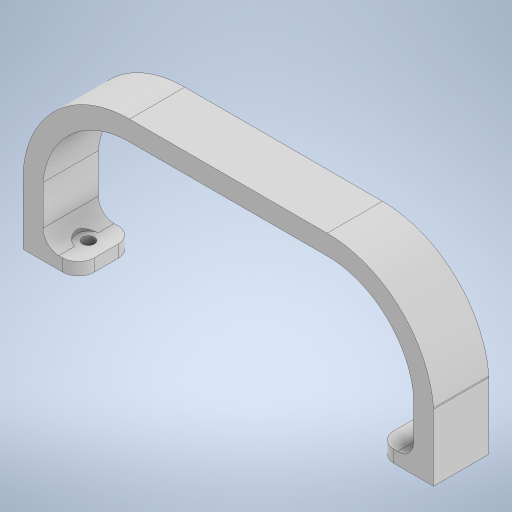
# Autodesk Inventor part: antenna_mount_v2
Saved by Autodesk Inventor 2024 (Build 280153000, 153)
## iProperties
Created: 2024-05-01
Part Number: antenna_mount_v2
Material: Generic
Document SubType Name: Modeling
Designer: Jacob
Density: 1 g/cm^3
Appearance: Default
Author: Jacob
## iProperties of the stored document antenna_mount_v2_3DPrint.ipt
Created: 2024-05-01
Part Number: antenna_mount_v2_3DPrint
Material: Generic
Document SubType Name: Modeling
Designer: Jacob
Density: 1 g/cm^3
Appearance: Default
Author: Jacob
Autodesk Inventor part; units mm, degrees
ref_plane "YZ Plane" through (0, 0, 0) normal (1, 0, 0) x (0, 1, 0)
sketch "Sketch11" plane through (0, 0, 0) normal (0, 0, 1) x (1, 0, 0)
  line L0 (25, -2.5) -> (-25, -2.5)
  line L1 (-25, -2.5) -> (-25, 2.5)
  line L2 (-25, 2.5) -> (25, 2.5)
  line L3 (25, 2.5) -> (25, -2.5)
  line L4 (25, -2.5) -> (-25, 2.5) construction
  line L5 (-25, -2.5) -> (25, 2.5) construction
  line L6 (0, 0) -> (-52.5, 0)
  line L7 (0, 0) -> (52.5, 0)
  circle A0 centre (25, -24.5) radius 24.5
  line L8 (52.5, 0) -> (52.5, -27.0879)
  circle A1 centre (25, -24.5) radius 27
  circle A2 centre (25, -24.5) radius 22
  line L9 (0, -2.5) -> (0, -42.1682)
  circle A3 centre (-25, -24.5) radius 24.5
  circle A4 centre (-25, -24.5) radius 27
  circle A5 centre (-25, -24.5) radius 22
  line L10 (-25, -24.5) -> (-52, -24.5)
  line L11 (-25, -24.5) -> (52.5, -24.5)
  point P0 (25, 0)
  point P1 (-47, -24.5)
  point P2 (47, -24.5)
  point P3 (52, -24.5)
  dimension "d43" = 49
  dimension "d39" = 50
  dimension "d40" = 5
  dimension "d41" = 52.5
  dimension "d42" = 52.5
  constraints: 24 end point, 5 horizontal, 4 coincident, 4 midpoint, 3 symmetric about line, 3 vertical, 2 centre point, 2 parallel, 2 point on line, 1 perpendicular, 1 vertical alignment, 13 other
  measures "d39" distance of L1.end L2.end
  measures "d40" distance of L0.end L1.end
  measures "d41" distance of L6.start L6.end
  measures "d42" distance of L6.start L7.end
extrude "Extrusion9" add sketch "Sketch11" along normal blind 12.5 contours L0 A0 L3 | L3 A0 L11 A2 | L0 A1 L7 A0 | L7 A1 L3 | L3 A1 L7 | L7 A1 L11 A0 | L0 A4 L6 L7 A1 | A1 L7 L6 A4 L2 | A4 L6 L1 | L1 L6 A4 | L0 A3 L6 A4 | A3 L0 L1 | A3 L10 A4 L6 | L1 A5 L10 A3
ref_plane "Work Plane1" through (-25, -39.5, 0) normal (0, -1, 0) x (1, 0, 0)
sketch "Sketch12" plane through (-25, -39.5, 0) normal (0, -1, 0) x (1, 0, 0)
  line L0 (25, 0) -> (25, 12.5)
  line L1 (50, 12.5) -> (0, 12.5) projected
  line L2 (25, 6.25) -> (0, 6.25)
  line L3 (0, 6.25) -> (50, 6.25)
  line L4 (0, 6.25) -> (5, 6.25)
  line L5 (5, 6.25) -> (5, 12.5)
  line L6 (5, 12.5) -> (0, 12.5)
  line L7 (0, 12.5) -> (0, 6.25)
  line L8 (5, 6.25) -> (0, 6.25)
  line L9 (0, 6.25) -> (0, 0)
  line L10 (0, 0) -> (5, 0)
  line L11 (5, 0) -> (5, 6.25)
  line L12 (50, 6.25) -> (45, 6.25)
  line L13 (45, 6.25) -> (45, 12.5)
  line L14 (45, 12.5) -> (50, 12.5)
  line L15 (50, 12.5) -> (50, 6.25)
  line L16 (50, 0) -> (72, 0) projected
  line L17 (50, 6.25) -> (45, 6.25)
  line L18 (45, 6.25) -> (45, 0)
  line L19 (45, 0) -> (50, 0)
  line L20 (50, 0) -> (50, 6.25)
  point P0 (50, 0)
  point P1 (45, 6.25)
  point P2 (45, 6.25)
  dimension "d47" = 25
  dimension "d48" = 50
  dimension "d49" = 5
  dimension "d50" = 5
  constraints: 38 end point, 8 parallel, 6 point on line, 5 horizontal, 4 perpendicular, 2 midpoint
  measures "d47" distance of L2.start L2.end
  measures "d48" distance of L2.end L3.end
  measures "d49" distance of L6.end L5.end
  measures "d50" distance of L13.end L14.end
extrude "Extrusion10" add sketch "Sketch12" against normal up to surface (37 mm away) contours L11 L10 L9 L2 | L2 L7 L1 L5 | L13 L1 L15 L3 | L3 L20 L19 L18
sketch "Sketch13" plane through (-25, -39.5, 0) normal (-1, 0, 0) x (0, 0, 1)
  line L0 (0, 0) -> (12.5, 0) projected
  line L1 (0, 0) -> (0, 37) projected
  line L2 (12.5, 0) -> (0, 0)
  line L3 (0, 0) -> (0, 3)
  line L4 (0, 3) -> (12.5, 3)
  line L5 (12.5, 3) -> (12.5, 0)
  line L6 (0, 0) -> (12.5, 0)
  line L7 (12.5, 0) -> (12.5, 3)
  line L8 (12.5, 3) -> (0, 3)
  line L9 (0, 3) -> (0, 0)
  point P0 (0, 39.5)
  dimension "d53" = 3
  constraints: 16 end point, 4 parallel, 2 horizontal, 2 perpendicular, 1 point on line
  measures "d53" distance of L2.end L3.end
extrude "Extrusion11" add sketch "Sketch13" along normal blind 8.75
sketch "Sketch14" plane through (25, -39.5, 12.5) normal (1, 0, 0) x (0, 0, -1)
  line L0 (0, 3) -> (12.5, 3) projected
  line L1 (12.5, 0) -> (0, 0)
  line L2 (0, 0) -> (0, 3)
  line L3 (0, 3) -> (12.5, 3)
  line L4 (12.5, 3) -> (12.5, 0)
  point P0 (12.5, 39.5)
  constraints: 8 end point, 2 parallel, 1 horizontal, 1 perpendicular
extrude "Extrusion12" add sketch "Sketch14" along normal blind 8.75
fillet "Fillet7" radius 2 4 edges at (-52, -24.5, 6.25) (-47, -24.5, 6.25) (47, -24.5, 6.25) (52, -24.5, 6.25)
fillet "Fillet9" radius 5 2 edges at (-33.75, -38, 0) (33.75, -38, 0)
sketch "Sketch15" plane through (-25, -39.5, 0) normal (0, -1, 0) x (1, 0, 0)
  circle A0 centre (53.75, 6.25) radius 1.4 projected
  circle A1 centre (-3.75, 6.25) radius 1.4 projected
  point P0 (25, 0)
extrude "Extrusion13" cut sketch "Sketch15" against normal blind 8.75
ref_plane "Work Plane3" through (30, -36.5, 12.5) normal (0, 1, 0) x (1, 0, 0)
sketch "Sketch16" plane through (30, -36.5, 12.5) normal (0, 1, 0) x (1, 0, 0)
  circle A0 centre (-58.75, 6.25) radius 1.4 projected
  circle A1 centre (-1.25, 6.25) radius 1.4 projected
  circle A2 centre (-58.75, 6.25) radius 2.5
  circle A3 centre (-1.25, 6.25) radius 2.5
  point P0 (-30, 12.5)
  dimension "d64" = 5
  dimension "d65" = 5
  constraints: 2 centre point, 2 coincident
  measures "d64" diameter of A2
  measures "d65" diameter of A3
extrude "Extrusion14" cut sketch "Sketch16" along normal blind 8.75 contours A0 | A1 | A2 | A3
sketch "Sketch17" plane through (0, 0, 12.5) normal (0, 0, 1) x (1, 0, 0)
  arc A0 (49.9199, -24.5) -> (51.9135, -22.34) centre (49.9199, -22.5) ccw projected
  arc A1 (51.9135, -22.34) -> (25, 2.5) centre (25, -24.5) ccw projected
  line L0 (25, 2.5) -> (-25, 2.5) projected
  arc A2 (-25, 2.5) -> (-51.9135, -22.34) centre (-25, -24.5) ccw projected
  arc A3 (-51.9135, -22.34) -> (-49.9199, -24.5) centre (-49.9199, -22.5) ccw projected
  line L1 (-49.9199, -24.5) -> (-48.9165, -24.5) projected
  arc A4 (-48.9165, -24.5) -> (-46.9235, -22.6667) centre (-48.9165, -22.5) ccw projected
  arc A5 (-25, -2.5) -> (-46.9235, -22.6667) centre (-25, -24.5) ccw projected
  line L2 (-25, -36.5) -> (-25, -2.5) projected
  line L3 (-25, -36.5) -> (-33.75, -36.5) projected
  line L4 (-33.75, -39.5) -> (-33.75, -36.5) projected
  line L5 (-20, -39.5) -> (-33.75, -39.5) projected
  line L6 (-20, -39.5) -> (-20, -2.5) projected
  line L7 (-20, -2.5) -> (20, -2.5) projected
  line L8 (20, -39.5) -> (20, -2.5) projected
  line L9 (33.75, -39.5) -> (20, -39.5) projected
  line L10 (33.75, -36.5) -> (33.75, -39.5) projected
  line L11 (25, -36.5) -> (33.75, -36.5) projected
  line L12 (25, -36.5) -> (25, -2.5) projected
  arc A6 (46.9235, -22.6667) -> (25, -2.5) centre (25, -24.5) ccw projected
  arc A7 (46.9235, -22.6667) -> (48.9165, -24.5) centre (48.9165, -22.5) ccw projected
  line L13 (48.9165, -24.5) -> (49.9199, -24.5) projected
  point P0 (0, 0)
extrude "Extrusion15" add sketch "Sketch17" along normal blind 1.5
fillet "Fillet11" radius 5 2 edges at (33.75, -38, 14) (-33.75, -38, 14)
ref_plane "Work Plane2" through (-25, -39.5, 0) normal (0, -1, 0) x (1, 0, 0)
sketch "Sketch18" plane through (-25, -39.5, 0) normal (0, -1, 0) x (1, 0, 0)
  line L0 (-26.9135, 14) -> (-26.9135, 0) projected
  line L1 (76.9135, 0) -> (50, 0) projected
  line L2 (-26.9135, 14) -> (76.9135, 14)
  line L3 (76.9135, 14) -> (76.9135, 0)
  line L4 (76.9135, 0) -> (-26.9135, 0)
  line L5 (-26.9135, 0) -> (-26.9135, 14)
  line L6 (76.9135, 0) -> (62.9135, 0)
  line L7 (62.9135, 0) -> (62.9135, 14)
  line L8 (62.9135, 14) -> (76.9135, 14)
  line L9 (76.9135, 14) -> (76.9135, 0)
  line L10 (-26.9135, 0) -> (-12.9135, 0)
  line L11 (-12.9135, 0) -> (-12.9135, 14)
  line L12 (-12.9135, 14) -> (-26.9135, 14)
  line L13 (-26.9135, 14) -> (-26.9135, 0)
  point P0 (25, 0)
  point P1 (-12.9135, 0)
  point P2 (-12.9135, 14)
  dimension "d73" = 14
  dimension "d74" = 14
  dimension "d75" = 14
  dimension "d76" = 14
  constraints: 24 end point, 6 parallel, 3 horizontal, 3 perpendicular
  measures "d73" distance of L7.end L8.end
  measures "d74" distance of L6.end L7.end
  measures "d75" distance of L12.end L11.end
  measures "d76" distance of L11.end L10.end
extrude "Extrusion16" add sketch "Sketch18" against normal up to surface (17.16 mm away) contours L2 L11 L4 L0 | L2 L3 L1 L7
sketch "Sketch19" plane through (-25, -39.5, 0) normal (0, -1, 0) x (1, 0, 0)
  arc A0 (-3.75, 14) -> (-8.75, 9) centre (-3.75, 9) ccw projected
  line L0 (-8.75, 5) -> (-8.75, 9) projected
  arc A1 (-8.75, 5) -> (-3.75, 0) centre (-3.75, 5) ccw projected
  line L1 (-3.75, 0) -> (5, 0) projected
  line L2 (5, 0) -> (5, 14) projected
  line L3 (-3.75, 14) -> (5, 14) projected
  circle A2 centre (-3.75, 6.25) radius 1.4 projected
  arc A3 (58.75, 9) -> (53.75, 14) centre (53.75, 9) ccw projected
  line L4 (45, 14) -> (53.75, 14) projected
  line L5 (45, 14) -> (45, 0) projected
  line L6 (45, 0) -> (53.75, 0) projected
  arc A4 (53.75, 0) -> (58.75, 5) centre (53.75, 5) ccw projected
  line L7 (58.75, 5) -> (58.75, 9) projected
  circle A5 centre (53.75, 6.25) radius 1.4 projected
  point P0 (25, 0)
extrude "Extrusion17" cut sketch "Sketch19" against normal blind 10
sketch "Sketch20" plane through (-25, -29.5, 0) normal (0, -1, 0) x (1, 0, 0)
  line L0 (0, 0) -> (0, 14) projected
  line L1 (5, 0) -> (0, 0) projected
  line L2 (5, 14) -> (5, 0) projected
  line L3 (0, 14) -> (5, 14) projected
  line L4 (45, 14) -> (50, 14) projected
  line L5 (50, 14) -> (50, 0) projected
  line L6 (45, 14) -> (50, 14) projected
  line L7 (45, 0) -> (45, 14) projected
  line L8 (50, 0) -> (45, 0) projected
  point P0 (25, 0)
extrude "Extrusion18" cut sketch "Sketch20" against normal up to surface (27 mm away)
sketch "Sketch21" plane through (-46.8937, -22.34, 14) normal (0, 1, 0) x (1, 0, 0)
  line L0 (0, 0) -> (0, 14) projected
  line L1 (0, 0) -> (8.9802, 0) projected
  line L2 (8.9802, 0) -> (8.9802, 14) projected
  line L3 (8.9802, 14) -> (0, 14) projected
  line L4 (93.7874, 14) -> (93.7874, 0) projected
  line L5 (93.7874, 14) -> (84.8072, 14) projected
  line L6 (84.8072, 14) -> (84.8072, 0) projected
  line L7 (84.8072, 0) -> (93.7874, 0) projected
  point P0 (46.8937, 14)
extrude "Extrusion19" cut sketch "Sketch21" against normal blind 14
sketch "Sketch22" plane through (-25, -39.5, 0) normal (0, -1, 0) x (1, 0, 0)
  line L0 (-21.8937, 0) -> (-12.9135, 0) projected
  line L1 (-21.8937, 14) -> (-21.8937, 0) projected
  line L2 (-12.9135, 14) -> (-21.8937, 14) projected
  line L3 (-12.9135, 0) -> (-12.9135, 14) projected
  line L4 (71.8937, 14) -> (62.9135, 14) projected
  line L5 (71.8937, 0) -> (71.8937, 14) projected
  line L6 (62.9135, 0) -> (71.8937, 0) projected
  line L7 (62.9135, 14) -> (62.9135, 0) projected
  circle A0 centre (67.4036, 7) radius 1.5
  circle A1 centre (-17.4036, 7) radius 1.5
  point P0 (25, 0)
  dimension "d85" = 3
  dimension "d86" = 3
  constraints: 2 centre point
  measures "d85" diameter of A0
  measures "d86" diameter of A1
extrude "Extrusion20" cut sketch "Sketch22" against normal blind 14 contours A0 | A1
fillet "Fillet12" radius 4 6 edges at (-46.8937, -36.34, 7) (46.8937, -36.34, 7) (37.9135, -37.92, 0) (37.9135, -37.92, 14) (-37.9135, -37.92, 0) (-37.9135, -37.92, 14)
sketch "Sketch23" plane through (-46.8937, -36.34, 14) normal (0, 1, 0) x (1, 0, 0)
  spline S0 degree 5 poles (4, 8.4177) (3.9037, 8.3844) (3.812, 8.3435) (3.7256, 8.296) (3.645, 8.2428) (3.5199, 8.1458) (3.472, 8.1043) (3.427, 8.0609) (3.3847, 8.0158) (3.3133, 7.9314) (3.2831, 7.8926) (3.2548, 7.8529) (3.2283, 7.8125) (3.1835, 7.7378) (3.1646, 7.7038) (3.1469, 7.6693) (3.1304, 7.6345) (3.0649, 7.4842) (3.0274, 7.3654) (3.0026, 7.2444) (2.9901, 7.1222) (2.9901, 6.8774) (3.0026, 6.7549) (3.0277, 6.6335) (3.0653, 6.5143) (3.1313, 6.3635) (3.148, 6.3284) (3.1659, 6.2938) (3.185, 6.2596) (3.2299, 6.1851) (3.2562, 6.1451) (3.2843, 6.1058) (3.3142, 6.0674) (3.3854, 5.9835) (3.4276, 5.9385) (3.4726, 5.8952) (3.5204, 5.8538) (3.6454, 5.7569) (3.7259, 5.7038) (3.8123, 5.6564) (3.9039, 5.6156) (4, 5.5823) knots 0 0 0 0 0 0 0.119868 0.119868 0.119868 0.119868 0.20161 0.20161 0.20161 0.20161 0.26807 0.26807 0.26807 0.26807 0.32231 0.32231 0.32231 0.32231 0.499998 0.499998 0.499998 0.499998 0.678246 0.678246 0.678246 0.678246 0.73283 0.73283 0.73283 0.73283 0.798663 0.798663 0.798663 0.798663 0.880271 0.880271 0.880271 0.880271 1 1 1 1 1 1 projected
  arc A0 (4, 5.5823) -> (4, 8.4177) centre (4.4901, 7) ccw projected
  circle A1 centre (4.4901, 7) radius 1.5 projected
  arc A2 (89.7874, 8.4177) -> (89.7874, 5.5823) centre (89.2973, 7) ccw projected
  spline S1 degree 7 poles (89.7874, 5.5823) (89.8562, 5.6061) (89.9228, 5.6335) (89.987, 5.6642) (90.0486, 5.698) (90.1076, 5.7346) (90.1636, 5.7736) (90.253, 5.843) (90.2879, 5.8721) (90.3214, 5.9022) (90.3536, 5.9332) (90.3844, 5.965) (90.4139, 5.9975) (90.6473, 6.2741) (90.7817, 6.5524) (90.8471, 6.8501) (90.8468, 7.1512) (90.7813, 7.4474) (90.6471, 7.7274) (90.4133, 8.0032) (90.3838, 8.0357) (90.353, 8.0674) (90.3209, 8.0983) (90.2874, 8.1284) (90.2525, 8.1574) (90.1632, 8.2266) (90.1072, 8.2656) (90.0483, 8.3022) (89.9867, 8.3359) (89.9226, 8.3666) (89.8561, 8.3939) (89.7874, 8.4177) knots 0 0 0 0 0 0 0 0 0.119884 0.119884 0.119884 0.119884 0.119884 0.119884 0.201637 0.201637 0.201637 0.201637 0.201637 0.201637 0.798638 0.798638 0.798638 0.798638 0.798638 0.798638 0.880256 0.880256 0.880256 0.880256 0.880256 0.880256 1 1 1 1 1 1 1 1 projected
  circle A3 centre (89.2973, 7) radius 1.5 projected
  arc A4 (3.5099, 4.1647) -> (3.5099, 9.8353) centre (4.4901, 7) ccw
  arc A5 (90.2775, 9.8353) -> (90.2775, 4.1647) centre (89.2973, 7) ccw
  spline S2 degree 5 poles (3.5099, 9.8353) (2.808, 9.5925) (2.1806, 9.1331) (1.7197, 8.4856) (1.2605, 7) (1.7198, 5.5144) (2.1806, 4.8669) (2.808, 4.4075) (3.5099, 4.1647) knots 0 0 0 0 0 0 0.500002 0.500002 0.500002 1 1 1 1 1 1
  spline S3 degree 5 poles (90.2775, 9.8353) (90.9794, 9.5926) (91.6069, 9.133) (92.0676, 8.4856) (92.527, 6.9999) (92.0676, 5.5145) (91.6065, 4.867) (90.9796, 4.4074) (90.2775, 4.1647) knots 0 0 0 0 0 0 0.500001 0.500001 0.500001 1 1 1 1 1 1
  point P0 (46.8937, 14)
  dimension "d90" = 1.5
  dimension "d91" = 1.5
  constraints: 4 point on circle, 4 vertical alignment, 2 centre point, 2 concentric, 4 other
  measures "d90" radial gap between concentric circles of A0 A4
  measures "d91" radial gap between concentric circles of A2 A5
extrude "Extrusion21" cut sketch "Sketch23" along normal blind 14
body "Solid2"
